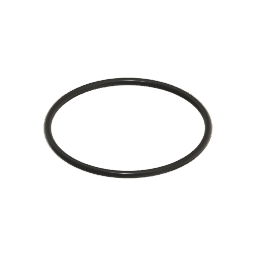
Zusammenbau v16 (Autodesk Fusion 360 archive; units mm, degrees)
design "O-Ring 42x46x2mm"
Autodesk Fusion 360 part; units mm, degrees
note: some values were not read from the file. Set by a fixed rule: the direction of a hole.
sketch "Skizze1" plane through (0, 0, 0) normal (0, 1, 0) x (1, 0, 0)
  line L0 (0, -65) -> (0, 31.1914) construction
  circle A0 centre (-21, -0.96) radius 1
  dimension "d1" = 2
  dimension "d2" = 21
  constraint vertical L0
  constraint coincident origin L0
  measures "d1" diameter of A0
  measures "d2" distance of L0 A0.centre
revolve "Drehen1" add sketch "Skizze1" angle 360 about axis through (0, 0, 65) along (0, 0, -1)
equation "d2 = ( 46 / 2 ) * 1 mm - 2 mm"

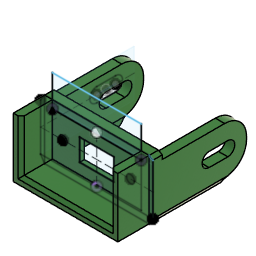
design "Sensorhalter"
Autodesk Fusion 360 part; units mm, degrees
sketch "Skizze1" plane through (0, 0, 0) normal (0, 0, 1) x (1, 0, 0)
  line L0 (-18, 30) -> (-18, 0)
  line L1 (-18, 0) -> (18, 0)
  line L2 (18, 0) -> (18, 30)
  line L3 (18, 30) -> (15, 30)
  line L4 (15, 30) -> (15, 3)
  line L5 (15, 3) -> (-15, 3)
  line L6 (-15, 3) -> (-15, 30)
  line L7 (-15, 30) -> (-18, 30)
  line L8 (0, 75) -> (0, -25) construction
  dimension "d1" = 3
  dimension "d2" = 3
  dimension "d3" = 36
  dimension "d4" = 30
  constraint vertical L0
  constraint perpendicular L0 L1
  constraint perpendicular L1 L2
  constraint perpendicular L2 L3
  constraint perpendicular L3 L4
  constraint perpendicular L4 L5
  constraint perpendicular L5 L6
  constraint perpendicular L0 L7
  constraint perpendicular L1 L8
  constraint symmetric L0 L2 L8
  constraint equal L0 L2
  measures "d1" distance of L6.end L0.start
  measures "d2" distance of L1 L5
  measures "d3" distance of L0 L2
  measures "d4" distance of L1 L7
extrude "Extrusion1" add sketch "Skizze1" along normal blind 15
sketch "Skizze2" plane through (-18, 0, 0) normal (-1, 0, 0) x (0, -1, 0)
  line L0 (-30, 0) -> (0, 0)
  line L1 (0, 0) -> (0, 15)
  line L2 (0, 15) -> (-30, 15)
  line L3 (-30, 15) -> (-30, 0)
  line L4 (-30, 7.5) -> (0, 7.5) construction
  line L5 (-24, 9.75) -> (-18, 9.75)
  line L6 (-18, 5.25) -> (-24, 5.25)
  arc A0 (-24, 9.75) -> (-24, 5.25) centre (-24, 7.5) ccw
  arc A1 (-18, 5.25) -> (-18, 9.75) centre (-18, 7.5) ccw
  dimension "d7" = 4.5
  dimension "d8" = 6
  dimension "d9" = 6
  constraint midpoint L3 L4.start
  constraint midpoint L1 L4.end
  constraint coincident L4 A0.centre
  constraint coincident L4 A1.centre
  constraint equal A0 A1
  constraint tangent L5 A0
  constraint tangent L5 A1
  constraint tangent L6 A1
  constraint tangent L6 A0
  measures "d7" diameter of A0
  measures "d8" distance of L3 A0.centre
  measures "d9" distance of A0.centre A1.centre
extrude "Extrusion2" cut sketch "Skizze2" against normal up to surface (36 mm away) contours L5 L6 A0 A1
fillet "Abrundung1" radius 7 4 edges at (-16.5, 30, 15) (16.5, 30, 15) (16.5, 30, 0) (-16.5, 30, 0)
sketch "Skizze3" plane through (0, 0, 0) normal (0, -1, 0) x (1, 0, 0)
  line L0 (-18, 0) -> (18, 0)
  line L1 (18, 0) -> (18, 15)
  line L2 (18, 15) -> (-18, 15)
  line L3 (-18, 15) -> (-18, 0)
  line L4 (18, 7.5) -> (-18, 7.5) construction
  circle A0 centre (10.8, 7.5) radius 1.25
  circle A1 centre (-10.8, 7.5) radius 1.25
  line L5 (14.25, 0.5) -> (-14.25, 0.5)
  line L6 (-14.25, 0.5) -> (-14.25, 14.5)
  line L7 (-14.25, 14.5) -> (14.25, 14.5)
  line L8 (14.25, 14.5) -> (14.25, 0.5)
  line L9 (18, 0) -> (-18, 0)
  line L10 (-18, 0) -> (-18, 15)
  line L11 (18, 16.3062) -> (18, 0)
  line L12 (0, 0) -> (0, 15) construction
  line L13 (16.75, -2) -> (-16.75, -2)
  line L14 (-16.75, -2) -> (-16.75, 17)
  line L15 (-16.75, 17) -> (16.75, 17)
  line L16 (16.75, 17) -> (16.75, -2)
  line L17 (18, 0) -> (16.75, -2)
  line L18 (-18, 0) -> (-16.75, -2)
  line L19 (-18, 15) -> (-16.75, 17)
  line L20 (16.75, 17) -> (18, 16.3062)
  line L21 (-5.5, 4) -> (5.5, 4)
  line L22 (5.5, 4) -> (5.5, 11)
  line L23 (5.5, 11) -> (-5.5, 11)
  line L24 (-5.5, 11) -> (-5.5, 4)
  dimension "d14" = 2.5
  dimension "d15" = 21.6
  dimension "d16" = 14
  dimension "d17" = 28.5
  dimension "d18" = 2.5
  dimension "d19" = 2.5
  dimension "d20" = 2.5
  dimension "d21" = 2.5
  dimension "d28" = 11
  dimension "d29" = 7
  constraint midpoint L1 L4.start
  constraint midpoint L3 L4.end
  constraint coincident L4 A0.centre
  constraint coincident L4 A1.centre
  constraint horizontal L5
  constraint vertical L6
  constraint horizontal L7
  constraint vertical L8
  constraint horizontal L9
  constraint vertical L10
  constraint vertical L11
  constraint coincident L2.end L3.start
  constraint coincident L0.end L1.start
  constraint equal A0 A1
  constraint coincident L12.start origin
  constraint symmetric A0.centre A1.centre L12
  constraint symmetric L4 L5 L7
  constraint symmetric L6 L8 L12
  constraint horizontal L13
  constraint vertical L14
  constraint horizontal L15
  constraint vertical L16
  constraint horizontal L21
  constraint vertical L22
  constraint horizontal L23
  constraint vertical L24
  constraint symmetric L12 L22 L24
  constraint symmetric L4 L21 L23
  measures "d14" diameter of A0
  measures "d15" distance of A0.centre A1.centre
  measures "d16" distance of L5.end L6.end
  measures "d17" distance of L5.start L5.end
  measures "d18" distance of L8 L16
  measures "d19" distance of L6 L14
  measures "d20" distance of L7 L15
  measures "d21" distance of L5 L13
  measures "d28" distance of L21.start L21.end
  measures "d29" distance of L21.end L22.end
extrude "Extrusion3" add sketch "Skizze3" against normal up to surface (3 mm away) contours L0 L9 L14 L18 | L0 L9 L13 L14 L16 | L2 L14 L19 | L0 L9 L16 L17 | L2 L14 L15 L16 | L2 L11 L16 L20
extrude "Extrusion4" cut sketch "Skizze3" against normal up to surface (3 mm away) contours A0 | A1
extrude "Extrusion5" cut sketch "Skizze3" against normal up to surface (3 mm away) contours L21 L22 L23 L24
chamfer "Fase2" distance 1.5 angle 45 4 edges at (0, 3, 4) (5.5, 3, 7.5) (0, 3, 11) (-5.5, 3, 7.5) measured on face at (-1.8333, 3, 15) measured on face at (-1.8333, 3, 15) measured on face at (-1.8333, 3, 15) measured on face at (-1.8333, 3, 15)
extrude "Extrusion6" add sketch "Skizze3" along normal blind 10 contours L0 L2 L9 L14 L16 | L0 L9 L13 L14 L16 | L2 L14 L15 L16
sketch "Skizze5" plane through (0, 0, 7.5) normal (0, -1, 0) x (1, 0, 0)
  line L0 (14.25, 7) -> (-14.25, 7)
  line L1 (-14.25, 7) -> (-14.25, 17)
  line L2 (-14.25, 17) -> (14.25, 17)
  line L3 (14.25, 17) -> (14.25, 7)
  point P0 (-14.25, 7)
  point P1 (14.25, 7)
  constraint horizontal L0
  constraint vertical L1
  constraint horizontal L2
  constraint vertical L3
  constraint coincident P0 L0.end
  constraint coincident L0.start L3.end
extrude "Extrusion8" cut sketch "Skizze5" along normal up to surface (10 mm away)
chamfer "Fase3" distance 1 angle 45 3 edges at (-14.25, -10, 8.75) (0, -10, 0.5) (14.25, -10, 8.75) measured on face at (-4.75, -10, -1.1667) measured on face at (-4.75, -10, -1.1667) measured on face at (-4.75, -10, -1.1667)
sketch "Skizze6" plane through (-18, 15, 7.5) normal (-1, 0, 0) x (0, -1, 0)
  line L0 (-9, 0) -> (-3, 0)
  point P0 (-6, 0)
  constraint horizontal L0
  constraint midpoint L0 P0
sketch "Skizze7" plane through (0, 3, 0) normal (0, 1, 0) x (-1, 0, 0)
  line L0 (15, 0) -> (15, 15)
  line L1 (15, 15) -> (18, 15)
  line L2 (18, 15) -> (16.75, 17)
  line L3 (16.75, 17) -> (-16.75, 17)
  line L4 (-16.75, 17) -> (-18, 16.3062)
  line L5 (-18, 16.3062) -> (-18, 15)
  line L6 (-18, 15) -> (-15, 15)
  line L7 (-15, 15) -> (-15, 0)
  line L8 (-15, 0) -> (-18, 0)
  line L9 (-18, 0) -> (-16.75, -2)
  line L10 (-16.75, -2) -> (16.75, -2)
  line L11 (16.75, -2) -> (18, 0)
  line L12 (18, 0) -> (15, 0)
  circle A0 centre (-10.8, 7.5) radius 1.25
  circle A1 centre (10.8, 7.5) radius 1.25
  line L13 (-7, 12.5) -> (7, 12.5)
  line L14 (7, 12.5) -> (7, 2.5)
  line L15 (7, 2.5) -> (-7, 2.5)
  line L16 (-7, 2.5) -> (-7, 12.5)
  line L17 (15, 0) -> (18, 0)
  line L18 (16.75, -2) -> (15, -2)
  line L19 (15, 0) -> (15, -2)
  line L20 (-15, 0) -> (-15, -2)
  line L21 (-16.75, -2) -> (-18, 0)
  constraint coincident L0.start L12.end
  constraint coincident L11.end L12.start
  constraint coincident L10.end L11.start
  constraint coincident L10 L18.end
  constraint parallel L10 L18
  constraint coincident L7.end L8.start
  constraint coincident L10 L20.end
  constraint perpendicular L10 L20
  constraint coincident L9.end L10.start
  constraint parallel L9 L21
extrude "Extrusion9" add sketch "Skizze7" along normal blind 20 contours L10 L11 L12 L17 L18 L19 | L8 L9 L10 L20 L21
fillet "Abrundung2" radius 2 3 edges at (-15.875, 23, -2) (16.5, 23, 0) (-16.5, 23, 0)

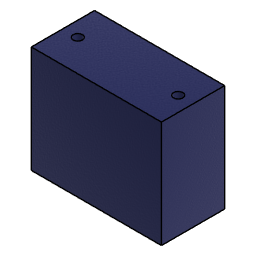
design "Sensor"
Autodesk Fusion 360 part; units mm, degrees
sketch "Skizze1" plane through (0, 0, 0) normal (0, 0, 1) x (1, 0, 0)
  line L0 (0, 0) -> (-28, 0)
  line L1 (-28, 0) -> (-28, 13.6)
  line L2 (-28, 13.6) -> (0, 13.6)
  line L3 (0, 13.6) -> (0, 0)
  line L4 (-28, 6.8) -> (0, 6.8) construction
  circle A0 centre (-24.8, 6.8) radius 1
  circle A1 centre (-3.2, 6.8) radius 1
  line L5 (-14, 13.6) -> (-14, 0) construction
  dimension "d1" = 13.6
  dimension "d2" = 28
  dimension "d5" = 2
  dimension "d6" = 2
  dimension "d7" = 21.6
  constraint horizontal L0
  constraint vertical L1
  constraint horizontal L2
  constraint vertical L3
  constraint coincident L0.start L3.end
  constraint midpoint L1 L4.start
  constraint midpoint L3 L4.end
  constraint coincident L4 A0.centre
  constraint coincident L4 A1.centre
  constraint midpoint L2 L5.start
  constraint midpoint L0 L5.end
  constraint symmetric A0.centre A1.centre L5
  measures "d1" distance of L0.start L2.end
  measures "d2" distance of L0.start L0.end
  measures "d5" diameter of A0
  measures "d6" diameter of A1
  measures "d7" distance of A0.centre A1.centre
extrude "Extrusion1" add sketch "Skizze1" along normal blind 23 contours L0 L1 L2 L3 | A0 | A1
extrude "Extrusion2" cut sketch "Skizze1" along normal up to surface (8 mm away) from surface at 15 contours A0 | A1

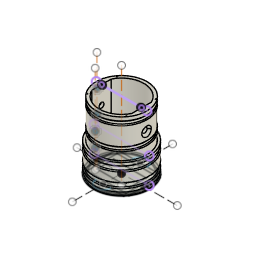
design "Gehäuse_unten"
Autodesk Fusion 360 part; units mm, degrees
sketch "Skizze1" plane through (0, 0, 0) normal (0, 0, 1) x (1, 0, 0)
  circle A0 centre (0, 0) radius 24.75
  circle A1 centre (0, 0) radius 21.75
  line L0 (-17.5, 13.5) -> (17.5, 13.5)
  line L1 (17.5, 13.5) -> (17.5, -13.5)
  line L2 (17.5, -13.5) -> (-17.5, -13.5)
  line L3 (-17.5, -13.5) -> (-17.5, 13.5)
  line L4 (-40, 0) -> (50, 0) construction
  line L5 (0, 45.7661) -> (0, -44.2339) construction
  line L6 (-18.4476, 16.5) -> (18.4476, 16.5)
  line L7 (20.5, 13.8677) -> (20.5, -13.8677)
  line L8 (18.4476, -16.5) -> (-18.4476, -16.5)
  line L9 (-20.5, -13.8677) -> (-20.5, 13.8677)
  arc A2 (6.5, 16.5) -> (-6.5, 16.5) centre (0, 16.5) ccw
  arc A3 (-6.6213, -16.5) -> (6.3787, -16.5) centre (-0.1213, -16.5) ccw
  arc A4 (-21.6357, 2.2272) -> (-21.6357, -2.2272) centre (-20.5, 0) ccw
  arc A5 (20.5, -2.5) -> (20.5, 2.5) centre (20.5, 0) ccw
  circle A6 centre (0, 0) radius 23 construction
  line L10 (-14.5, -7.5) -> (14.5, -7.5)
  line L11 (14.5, -7.5) -> (14.5, 7.5)
  line L12 (14.5, 7.5) -> (-14.5, 7.5)
  line L13 (-14.5, 7.5) -> (-14.5, -7.5)
  circle A7 centre (0, 0) radius 22.75
  dimension "d1" = 49.5
  dimension "d3" = 3
  dimension "d4" = 27
  dimension "d5" = 35
  dimension "d6" = 3
  dimension "d7" = 3
  dimension "d8" = 3
  dimension "d9" = 3
  dimension "d18" = 46
  dimension "d19" = 29
  dimension "d20" = 15
  dimension "d43" = 45.5
  constraint coincident A0.centre A1.centre
  constraint horizontal L0
  constraint vertical L1
  constraint horizontal L2
  constraint vertical L3
  constraint parallel L2 L4
  constraint symmetric L0 L2 L4
  constraint vertical L5
  constraint symmetric L1 L3 L5
  constraint coincident A0.centre L5
  constraint coincident A0.centre L4
  constraint horizontal L6
  constraint vertical L7
  constraint horizontal L8
  constraint vertical L9
  constraint equal A2 A3
  constraint coincident L6 A2.end
  constraint coincident L6 A2.start
  constraint coincident L8 A3.end
  constraint coincident L8 A3.start
  constraint coincident A0 L8.end
  constraint coincident L8 A3.centre
  constraint coincident A0 L9.start
  constraint coincident A0 L9.end
  constraint coincident A0 L6.start
  constraint coincident L6 A2.centre
  constraint coincident A0 L7.start
  constraint coincident A0 L6.end
  constraint coincident A0 L7.end
  constraint coincident A0 L8.start
  constraint midpoint L9 A4.centre
  constraint midpoint L7 A5.centre
  constraint equal A4 A5
  constraint coincident A1 A4.start
  constraint coincident A1 A4.end
  constraint coincident L7 A5.end
  constraint coincident L7 A5.start
  constraint concentric A0 A6
  constraint tangent A5 A6
  constraint tangent A2 A6
  constraint horizontal L10
  constraint vertical L11
  constraint horizontal L12
  constraint vertical L13
  constraint symmetric L5 L11 L13
  constraint symmetric L4 L10 L12
  constraint concentric A1 A7
  measures "d1" diameter of A0
  measures "d3" distance of A0 A1
  measures "d4" distance of L0.start L2.end
  measures "d5" distance of L0.start L0.end
  measures "d6" distance of L3 L9
  measures "d7" distance of L1 L7
  measures "d8" distance of L0 L6
  measures "d9" distance of L2 L8
  measures "d18" diameter of A6
  measures "d19" distance of L10.start L10.end
  measures "d20" distance of L10.end L11.end
  measures "d43" diameter of A7
extrude "Extrusion1" add sketch "Skizze1" along normal blind 60 contours A0 L7 A5 A7 | A0 L6 L7 A7 | A0 L7 L8 A7 | A0 L6 A2 A7 | A1 L7 A5 A7 | A1 L0 L1 L6 L7 A7 | A0 L8 A3 A7 | A1 L1 L2 L7 L8 A7 | A1 L7 A5 A7 | A0 L6 L9 A7 | A1 L6 A2 A7 | A1 A5 A7 | A5 A7 | A0 L8 L9 A7 | A1 L8 A3 A7 | A0 L9 A4 A7 | A1 L6 A2 A7 | A1 L0 L3 L6 L9 A7 | A2 A7 | A1 A2 A7 | A1 L2 L3 L8 L9 A7 | A1 L8 A3 A7 | A1 A3 A7 | A3 A7 | A1 L9 A4 A7 | A1 L9 A4 A7 | A4 A7 | A1 A4 A7
extrude "Extrusion2" add sketch "Skizze1" along normal blind 3 contours A1 L1 L7 | A1 L7 A5 | A1 L7 A5 | A1 L6 A2 | A1 L0 L6 | A1 L7 A5 | A1 L0 L1 L2 L3 | A1 L2 L8 | A1 L8 A3 | A1 L6 A2 | A1 L6 A2 | A1 L8 A3 | A1 L8 A3 | A1 L9 | A1 L3 L9 | L10 L11 L12 L13
chamfer "Fase1" distance 3 angle 12 1 edges at (-23.0751, -8.95, 0) measured on face at (24.627, -2.4643, 20)
extrude "Extrusion3" cut sketch "Skizze1" along normal up to surface (3 mm away) contours L10 L11 L12 L13
extrude "Extrusion4" add sketch "Skizze1" along normal up to surface (60 mm away) contours A1 L7 A5 | A1 L7 A5 | A1 L7 A5 | A1 L9
chamfer "Fase2" distance 1.5 angle 45 4 edges at (0, -7.5, 3) (-14.5, 0, 3) (0, 7.5, 3) (14.5, 0, 3) measured on face at (-0.5022, -12.2326, 3) measured on face at (-0.5022, -12.2326, 3) measured on face at (-0.5022, -12.2326, 3) measured on face at (-0.5022, -12.2326, 3)
sketch "Skizze2" plane through (-20.5, 0, 0) normal (1, 0, 0) x (0, 1, 0)
  line L0 (-7.2672, 3) -> (7.2672, 3)
  line L1 (7.2672, 3) -> (7.2672, 60)
  line L2 (7.2672, 60) -> (-7.2672, 60)
  line L3 (-7.2672, 60) -> (-7.2672, 3)
  line L4 (7.2672, 3) -> (12.9156, 3)
  line L5 (13.5, 3) -> (12.9156, 3)
  line L6 (13.5, 3) -> (21.75, 3)
  line L7 (13.5, 3) -> (12.9156, 3)
  line L8 (7.2672, 3) -> (12.9156, 3)
  line L9 (7.2672, 3) -> (-7.2672, 3)
  line L10 (-12.9156, 3) -> (-7.2672, 3)
  line L11 (-12.9156, 3) -> (-13.5, 3)
  line L12 (-21.75, 3) -> (-13.5, 3)
  line L13 (-12.9156, 3) -> (-13.5, 3)
  line L14 (-12.9156, 3) -> (-7.2672, 3)
  line L15 (-7.2672, 3) -> (7.2672, 3)
  line L16 (-9, 3) -> (9, 3)
  line L17 (9, 3) -> (-9, 3)
  line L18 (-21.75, 60) -> (-13.5, 60)
  line L19 (-13.5, 60) -> (-12.9156, 60)
  line L20 (-12.9156, 60) -> (-7.2672, 60)
  line L21 (-7.2672, 60) -> (7.2672, 60)
  line L22 (7.2672, 60) -> (12.9156, 60)
  line L23 (12.9156, 60) -> (13.5, 60)
  line L24 (13.5, 60) -> (21.75, 60)
  line L25 (13.5, 60) -> (12.9156, 60)
  line L26 (7.2672, 60) -> (12.9156, 60)
  line L27 (7.2672, 60) -> (-7.2672, 60)
  line L28 (-12.9156, 60) -> (-7.2672, 60)
  line L29 (-12.9156, 60) -> (-13.5, 60)
  line L30 (24.75, 60) -> (-24.75, 60)
  circle A0 centre (0, 44) radius 2.25
  line L31 (0, 60) -> (0, 3) construction
  dimension "d30" = 4.5
  dimension "d31" = 41
  constraint midpoint L21 L31.start
  constraint coincident A0.centre L31
  measures "d30" diameter of A0
  measures "d31" distance of L0 A0.centre
extrude "Extrusion5" cut sketch "Skizze2" along normal blind 110 and the other way blind 40 contours A0
hole "Bohrung1" at (-0.1213, -16.5, 0) at (20.5, 0, 0) at (0, 16.5, 0) at (-20.5, 0, 0) direction (0, 0, 1) diameter 2 depth 8 tip angle 118
sketch "Skizze4" plane through (0, 0, 3) normal (0, 0, 1) x (-1, 0, 0)
  arc A0 (-20.5, -1) -> (-20.5, 1) centre (-20.5, 0) ccw
  line L0 (-20.5, -1) -> (-20.5, -7.2672)
  arc A1 (-20.5, -7.2672) -> (-17.5, -12.9156) centre (0, 0) ccw
  arc A2 (-17.5, -12.9156) -> (-17.0532, -13.5) centre (0, 0) ccw
  arc A3 (-17.0532, -13.5) -> (17.0532, -13.5) centre (0, 0) ccw
  arc A4 (17.0532, -13.5) -> (17.5, -12.9156) centre (0, 0) ccw
  arc A5 (17.5, -12.9156) -> (20.5, -7.2672) centre (0, 0) ccw
  line L1 (20.5, -7.2672) -> (20.5, -1)
  arc A6 (20.5, 1) -> (20.5, -1) centre (20.5, 0) ccw
  line L2 (20.5, 1) -> (20.5, 7.2672)
  arc A7 (20.5, 7.2672) -> (17.5, 12.9156) centre (0, 0) ccw
  arc A8 (17.5, 12.9156) -> (17.0532, 13.5) centre (0, 0) ccw
  arc A9 (17.0532, 13.5) -> (-17.0532, 13.5) centre (0, 0) ccw
  arc A10 (-17.0532, 13.5) -> (-17.5, 12.9156) centre (0, 0) ccw
  arc A11 (-17.5, 12.9156) -> (-20.5, 7.2672) centre (0, 0) ccw
  line L3 (-20.5, 7.2672) -> (-20.5, 1)
  circle A12 centre (0, -16.5) radius 1
  circle A13 centre (0.1213, 16.5) radius 1
  line L4 (-16, 9) -> (16, 9)
  line L5 (16, 9) -> (16, -9)
  line L6 (16, -9) -> (-16, -9)
  line L7 (-16, -9) -> (-16, 9)
  line L8 (20.5, -2.25) -> (20.5, 2.25)
  line L9 (20.5, 1) -> (20.5, 0)
  line L10 (20.5, 0) -> (20.5, -1)
  line L11 (20.5, -1) -> (20.5, -7.2672)
  line L12 (20.5, -7.2672) -> (20.5, 7.2672)
  line L13 (20.5, 7.2672) -> (20.5, 1)
  arc A14 (17.5, -12.9156) -> (20.5, -7.2672) centre (0, 0) ccw
  arc A15 (17.5, -12.9156) -> (20.5, -7.2672) centre (0, 0) ccw
  arc A16 (-17.0532, -13.5) -> (17.0532, -13.5) centre (0, 0) ccw
  arc A17 (-17.0532, -13.5) -> (17.0532, -13.5) centre (0, 0) ccw
  arc A18 (20.5, 7.2672) -> (17.5, 12.9156) centre (0, 0) ccw
  arc A19 (20.5, 7.2672) -> (17.5, 12.9156) centre (0, 0) ccw
  arc A20 (-20.5, -7.2672) -> (-17.5, -12.9156) centre (0, 0) ccw
  arc A21 (-20.5, -7.2672) -> (-17.5, -12.9156) centre (0, 0) ccw
  line L14 (-20.5, 2.25) -> (-20.5, -2.25)
  line L15 (-20.5, -1) -> (-20.5, 0)
  line L16 (-20.5, 0) -> (-20.5, 1)
  line L17 (-20.5, 1) -> (-20.5, 7.2672)
  line L18 (-20.5, 7.2672) -> (-20.5, -7.2672)
  line L19 (-20.5, -7.2672) -> (-20.5, -1)
  arc A22 (-17.5, 12.9156) -> (-20.5, 7.2672) centre (0, 0) ccw
  arc A23 (-17.5, 12.9156) -> (-20.5, 7.2672) centre (0, 0) ccw
  arc A24 (17.0532, 13.5) -> (-17.0532, 13.5) centre (0, 0) ccw
  arc A25 (17.0532, 13.5) -> (-17.0532, 13.5) centre (0, 0) ccw
  circle A26 centre (0, -16.5) radius 1
  circle A27 centre (0.1213, 16.5) radius 1
  circle A28 centre (0, 0) radius 20
  line L20 (18, -8.7178) -> (18, 8.7178)
  line L21 (-18, -8.7178) -> (-18, 8.7178)
  point P0 (20.5, -21.75)
  dimension "d47" = 40
  dimension "d48" = 36
  constraint concentric A20 A28
  constraint coincident A28 L20.start
  constraint coincident A28 L20.end
  constraint vertical L20
  constraint coincident A28 L21.start
  constraint coincident A28 L21.end
  constraint vertical L21
  constraint equal L20 L21
  measures "d47" diameter of A28
  measures "d48" distance of L20 L21
extrude "Extrusion7" add sketch "Skizze4" along normal up to surface (57 mm away) contours A0 L14 L15 L16 L18 A28 | A0 L0 A1 A2 A3 A4 A5 L1 A6 L8 L11 L12 A14 A15 A16 A17 A20 A21 L14 L18 L19 A28 | A0 A28 | A0 A28 L21 | A0 A6 L2 A7 A8 A9 A10 A11 L3 L8 L12 L13 A18 A19 L14 L17 L18 A22 A23 A24 A25 A28 | A6 A28 L20 | A6 L8 L9 L10 L12 A28 | A6 A28
extrude "Extrusion6" cut sketch "Skizze1" along normal up to surface (34 mm away) from surface at 26 contours A0 L7 A5 A7 | A0 L6 L7 A7 | A0 L7 L8 A7 | A0 L6 A2 A7 | A0 L8 A3 A7 | A0 L6 L9 A7 | A5 A7 | A0 L8 L9 A7 | A0 L9 A4 A7 | A2 A7 | A3 A7 | A4 A7
extrude "Extrusion8" cut sketch "Skizze2" along normal blind 55 contours A0
sketch "Skizze3" plane through (0, 0, 0) normal (0, 1, 0) x (1, 0, 0)
  line L0 (-17.0532, -60) -> (-17.5, -60)
  line L1 (-17.5, -60) -> (-17.0532, -60)
  line L2 (17.0532, -60) -> (17.5, -60)
  line L3 (17.5, -60) -> (17.0532, -60)
  line L4 (-22.1, -83.0309) -> (-22.1, 7) construction
  line L5 (0, -84) -> (0, 9) construction
  circle A0 centre (-22.1, -55) radius 1.1
  circle A1 centre (-22.1, -35) radius 1.1
  line L6 (-22.75, -60) -> (22.75, -60)
  line L7 (17.5, -60) -> (17.0532, -60)
  line L8 (17.5, -60) -> (17.0532, -60)
  line L9 (-17.0532, -60) -> (-17.5, -60)
  line L10 (-18, -60) -> (18, -60)
  line L11 (-18, -60) -> (18, -60)
  line L12 (-17.0532, -60) -> (-17.5, -60)
  circle A2 centre (-23.7, -21) radius 1.6
  circle A3 centre (-23.7, -8) radius 1.6
  line L13 (-23.7, 9.1317) -> (-23.7, -70) construction
  line L14 (24.75, -3) -> (-24.75, -3)
  line L15 (24.75, -26) -> (-24.75, -26)
  dimension "d38" = 22.1
  dimension "d39" = 2.2
  dimension "d56" = 3.2
  dimension "d57" = 5
  dimension "d58" = 5
  dimension "d59" = 23.7
  constraint vertical L5
  constraint coincident L4 A0.centre
  constraint coincident L4 A1.centre
  constraint equal A0 A1
  constraint vertical L13
  constraint coincident A3.centre L13
  constraint coincident A2.centre L13
  constraint equal A2 A3
  measures "d38" distance of L4 L5
  measures "d39" diameter of A0
  measures "d56" diameter of A2
  measures "d57" distance of A3.centre L14
  measures "d58" distance of A2.centre L15
  measures "d59" distance of L5 L13
revolve "Drehen2" cut sketch "Skizze3" angle 360 about axis through (0, 0, 84) along (0, 0, -1) contours A0 | A1
revolve "Drehen3" cut sketch "Skizze3" angle 360 about axis through (0, 0, 84) along (0, 0, -1) contours A2 | A3
fillet "Abrundung1" radius 0.75 8 edges at (-21.2104, -8.2268, 55.8874) (-21.2104, 8.2268, 54.1126) (-21.2104, -8.2268, 35.8874) (-21.2104, 8.2268, 34.1126) (-23.0751, -8.95, 22.2073) (-23.0751, 8.95, 19.7927) (-23.0751, -8.95, 9.2073) (-23.0751, 8.95, 6.7927)
chamfer "Fase4" distance 2 angle 45 2 edges at (-22.6385, -2.25, 44) (22.6385, -2.25, 44)
equation "d38 = ( 45.5 / 2 ) * 1 mm - 0.65 mm"
equation "d59 = ( 49 / 2 ) * 1 mm - 0.8 mm"

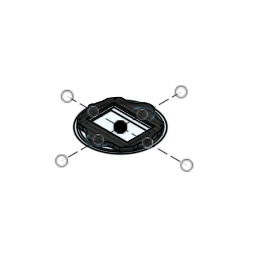
design "Glasträger"
Autodesk Fusion 360 part; units mm, degrees
sketch "Skizze1" plane through (0, 0, 0) normal (0, 0, 1) x (1, 0, 0)
  circle A0 centre (0, 0) radius 24.75
  circle A1 centre (0, 0) radius 21.75
  line L0 (-17.5, 13.5) -> (17.5, 13.5)
  line L1 (17.5, 13.5) -> (17.5, -13.5)
  line L2 (17.5, -13.5) -> (-17.5, -13.5)
  line L3 (-17.5, -13.5) -> (-17.5, 13.5)
  line L4 (-40, 0) -> (50, 0) construction
  line L5 (0, 45.7661) -> (0, -44.2339) construction
  line L6 (-16.0234, 16.5) -> (16.0234, 16.5)
  line L7 (20.5, 10.4283) -> (20.5, -10.4283)
  line L8 (16.0234, -16.5) -> (-16.0234, -16.5)
  line L9 (-20.5, -10.4283) -> (-20.5, 10.4283)
  arc A2 (6.5, 16.5) -> (-6.5, 16.5) centre (0, 16.5) ccw
  arc A3 (-6.6213, -16.5) -> (6.3787, -16.5) centre (-0.1213, -16.5) ccw
  arc A4 (-21.6357, 2.2272) -> (-21.6357, -2.2272) centre (-20.5, 0) ccw
  arc A5 (21.6357, -2.2272) -> (21.6357, 2.2272) centre (20.5, 0) ccw
  circle A6 centre (0, 0) radius 23
  line L10 (-14.5, -7.5) -> (14.5, -7.5)
  line L11 (14.5, -7.5) -> (14.5, 7.5)
  line L12 (14.5, 7.5) -> (-14.5, 7.5)
  line L13 (-14.5, 7.5) -> (-14.5, -7.5)
  line L14 (-15.5, 10.5) -> (15.5, 10.5)
  line L15 (15.5, 10.5) -> (15.5, -10.5)
  line L16 (15.5, -10.5) -> (-15.5, -10.5)
  line L17 (-15.5, -10.5) -> (-15.5, 10.5)
  dimension "d1" = 49.5
  dimension "d3" = 3
  dimension "d4" = 27
  dimension "d5" = 35
  dimension "d6" = 3
  dimension "d7" = 3
  dimension "d8" = 3
  dimension "d9" = 3
  dimension "d18" = 46
  dimension "d19" = 29
  dimension "d20" = 15
  dimension "d27" = 3
  dimension "d28" = 3
  dimension "d29" = 2
  dimension "d30" = 2
  dimension "d40" = 33
  constraint coincident A0.centre A1.centre
  constraint horizontal L0
  constraint vertical L1
  constraint horizontal L2
  constraint vertical L3
  constraint parallel L2 L4
  constraint symmetric L0 L2 L4
  constraint vertical L5
  constraint symmetric L1 L3 L5
  constraint coincident A0.centre L5
  constraint coincident A0.centre L4
  constraint horizontal L6
  constraint vertical L7
  constraint horizontal L8
  constraint vertical L9
  constraint equal A2 A3
  constraint coincident L6 A2.end
  constraint coincident L6 A2.start
  constraint coincident L8 A3.end
  constraint coincident L8 A3.start
  constraint coincident L8 A3.centre
  constraint coincident L6 A2.centre
  constraint equal A4 A5
  constraint coincident A1 A4.start
  constraint coincident A1 A4.end
  constraint concentric A0 A6
  constraint tangent A5 A6
  constraint tangent A2 A6
  constraint horizontal L10
  constraint vertical L11
  constraint horizontal L12
  constraint vertical L13
  constraint symmetric L5 L11 L13
  constraint symmetric L4 L10 L12
  constraint coincident A6 L7.end
  constraint coincident L7 A5.centre
  constraint coincident A6 L8.start
  constraint coincident A6 L9.start
  constraint coincident L9 A4.centre
  constraint coincident A6 L8.end
  constraint coincident A6 L6.start
  constraint coincident A6 L9.end
  constraint coincident A6 L6.end
  constraint coincident A6 L7.start
  constraint coincident A1 A5.end
  constraint coincident A1 A5.start
  constraint horizontal L14
  constraint vertical L15
  constraint horizontal L16
  constraint vertical L17
  measures "d1" diameter of A0
  measures "d3" distance of A0 A1
  measures "d4" distance of L0.start L2.end
  measures "d5" distance of L0.start L0.end
  measures "d6" distance of L3 L9
  measures "d7" distance of L1 L7
  measures "d8" distance of L0 L6
  measures "d9" distance of L2 L8
  measures "d18" diameter of A6
  measures "d19" distance of L10.start L10.end
  measures "d20" distance of L10.end L11.end
  measures "d27" distance of L0 L14
  measures "d28" distance of L2 L16
  measures "d29" distance of L1 L15
  measures "d30" distance of L3 L17
  measures "d40" distance of L6 L8
extrude "Extrusion5" add sketch "Skizze1" along normal blind 3 contours A1 L7 | A1 A5 | A1 L1 L7 | A1 L0 L1 L6 L7 A6 | A1 L1 L2 L7 L8 A6 | A1 L0 L6 | A1 L2 L8 | A1 L0 L3 L6 L9 A6 | A1 A2 | A1 A3 | A1 L2 L3 L8 L9 A6 | A1 L6 A2 | A1 L3 L9 | A1 L8 A3 | A1 L9 | A1 A4 picked at (0.4894, 18.2335) picked at (-0.6234, -18.2297)
extrude "Extrusion6" add sketch "Skizze1" along normal up to surface (1.5 mm away) from surface at 1.5 contours A1 L0 L1 L2 L3
hole "Bohrung1" at (0, 16.5, 0) at (20.5, 0, 0) at (-0.1213, -16.5, 0) at (-20.5, 0, 0) direction (0, 0, 1) diameter 2.5 end through all
fillet "Abrundung1" radius 7 4 edges at (-6.6213, -16.5, 1.5) (6.3787, -16.5, 1.5) (6.5, 16.5, 1.5) (-6.5, 16.5, 1.5)

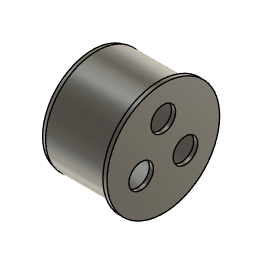
design "Stopfen DN50 mod"
Autodesk Fusion 360 part; units mm, degrees
sketch "Skizze1" plane through (0, 0, 0) normal (0, 0, 1) x (1, 0, 0)
  line L0 (0, 0) -> (0, 27.5)
  line L1 (0, 27.5) -> (-2, 27.5)
  line L2 (-2, 27.5) -> (-2, 25)
  line L3 (-2, 25) -> (-32.5, 25)
  line L4 (-32.5, 25) -> (-34.5, 24.4641)
  line L5 (-34.5, 24.4641) -> (-34.5, 23)
  line L6 (-34.5, 23) -> (-2, 23)
  line L7 (-2, 23) -> (-2, 0)
  line L8 (-2, 0) -> (0, 0)
  dimension "d2" = 27.5
  dimension "d3" = 32.5
  dimension "d4" = 2
  dimension "d5" = 23
  dimension "d6" = 25
  dimension "d7" = 15
  dimension "d8" = 2
  constraint coincident L0.start L8.end
  constraint vertical L0
  constraint perpendicular L0 L1
  constraint perpendicular L1 L2
  constraint perpendicular L2 L3
  constraint perpendicular L3 L5
  constraint perpendicular L5 L6
  constraint perpendicular L6 L7
  constraint perpendicular L0 L8
  constraint collinear L2 L7
  measures "d2" distance of L0.start L0.end
  measures "d3" distance of L5.end L6.end
  measures "d4" distance of L0.end L1.end
  measures "d5" distance of L6.end L7.end
  measures "d6" distance of L3 L8
  measures "d7" angle of L3 L4
  measures "d8" distance of L3.end L5
revolve "Drehen1" add sketch "Skizze1" angle 360 about axis through (1.75, 0, 0) along (1, 0, 0)
sketch "Skizze3" plane through (0, 0, 0) normal (1, 0, 0) x (0, 1, 0)
  circle A0 centre (0, 0) radius 27.5
  circle A1 centre (-10.8253, -6.25) radius 6
  circle A2 centre (0, 12.5) radius 6
  circle A3 centre (10.8253, -6.25) radius 6
  line L0 (0, 0) -> (0, 27.5) construction
  line L1 (0, 0) -> (23.8157, -13.75) construction
  line L2 (0, 0) -> (-23.8157, -13.75) construction
  circle A4 centre (0, 0) radius 12.5 construction
  circle A5 centre (0, 0) radius 23
  circle A6 centre (0, 0) radius 23
  dimension "d9" = 120
  dimension "d10" = 120
  dimension "d11" = 12
  dimension "d12" = 25
  constraint coincident A0.centre L0.start
  constraint coincident A0 L0.end
  constraint vertical L0
  constraint coincident A0 L1.end
  constraint coincident A0 L2.end
  constraint coincident A2.centre L0
  constraint coincident A1.centre L2
  constraint coincident A3.centre L1
  constraint equal A2 A3
  constraint equal A1 A2
  constraint concentric A0 A4
  constraint coincident A2.centre A4
  constraint coincident A3.centre A4
  constraint coincident A1.centre A4
  measures "d9" angle of L0 L1
  measures "d10" angle of L0 L2
  measures "d11" diameter of A3
  measures "d12" diameter of A4
extrude "Extrusion1" cut sketch "Skizze3" against normal up to surface (2 mm away) contours A1 | A2 | A3
equation "d2 = ( 55 / 2 ) * 1 mm"
equation "d5 = ( 46 / 2 ) * 1 mm"
equation "d6 = ( 50 / 2 ) * 1 mm"

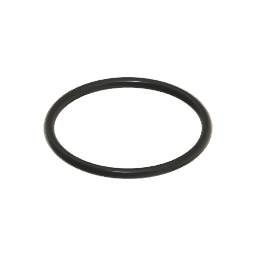
design "O-Ring 44x50x3mm"
Autodesk Fusion 360 part; units mm, degrees
sketch "Skizze1" plane through (0, 0, 0) normal (0, 1, 0) x (1, 0, 0)
  line L0 (0, -65) -> (0, 31.1914) construction
  circle A0 centre (-22, -0.96) radius 1.5
  dimension "d1" = 3
  dimension "d2" = 22
  constraint vertical L0
  constraint coincident origin L0
  measures "d1" diameter of A0
  measures "d2" distance of L0 A0.centre
revolve "Drehen1" add sketch "Skizze1" angle 360 about axis through (0, 0, 65) along (0, 0, -1)
equation "d2 = ( 50 / 2 ) * 1 mm - 3 mm"
